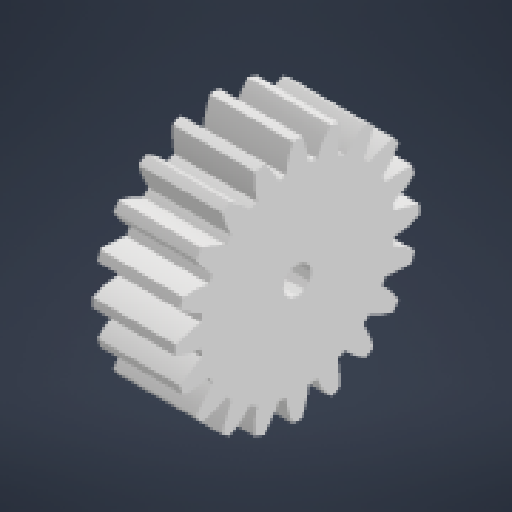
# Autodesk Inventor part: gear base
Saved by Autodesk Inventor 2024 (Build 280153000, 153)
## iProperties
Created: 2023-06-18
Part Number: gear base
Material: 일반
Document SubType Name: Modeling
Designer: 6gioc
Density: 1 g/cm^3
Appearance: 기본값
Mass: 18.4173 g
Surface Area: 64.8301 cm^2
Volume: 18.4173 cm^3
Author: 6gioc
Autodesk Inventor part; units mm, degrees
ref_plane "YZ Plane" through (0, 0, 0) normal (1, 0, 0) x (0, 1, 0)
ref_plane "XZ Plane" through (0, 0, 0) normal (0, 1, 0) x (-1, 0, 0)
ref_plane "XY Plane" through (0, 0, 0) normal (0, 0, 1) x (1, 0, 0)
sketch "스케치1" plane through (0, 0, 0) normal (1, 0, 0) x (0, 1, 0)
  circle A0 centre (0, 0) radius 22.155
  circle A1 centre (0, 0) radius 2.5
  line L0 (2.5, 0) -> (2.1651, -1.25)
  line L1 (2.1651, -1.25) -> (1.25, -2.1651)
  line L2 (1.25, -2.1651) -> (0, -2.5)
  line L3 (0, -2.5) -> (-1.25, -2.1651)
  line L4 (-1.25, -2.1651) -> (-2.1651, -1.25)
  line L5 (-2.1651, -1.25) -> (-2.5, 0)
  line L6 (-2.5, 0) -> (-2.1651, 1.25)
  line L7 (-2.1651, 1.25) -> (-1.25, 2.1651)
  line L8 (-1.25, 2.1651) -> (0, 2.5)
  line L9 (0, 2.5) -> (1.25, 2.1651)
  line L10 (1.25, 2.1651) -> (2.1651, 1.25)
  line L11 (2.1651, 1.25) -> (2.5, 0)
  dimension "d4" = 5
  dimension "d0" = 44.31
  constraints: 24 end point, 4 coincident, 1 centre point, 1 horizontal alignment, 27 other
  measures "d0" diameter of A0
extrude "돌출1" add sketch "스케치1" along normal blind 15 contours A0 | L11 A1 | A1 L0 | L10 A1 | A1 L1 | L9 A1 | A1 L2 | L8 A1 | A1 L3 | L7 A1 | A1 L4 | L6 A1 | A1 L5
spur gear teeth "스퍼 기어1" teeth 20 pitch diameter 40 tip diameter 44 root diameter 35 face width 15 trims to tip circle yes start plane through (15, 0, 0) normal (1, 0, 0) x (0, 1, 0)
